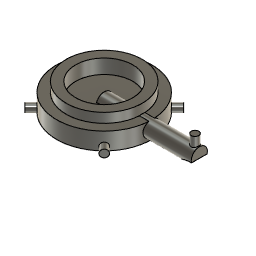
base v4 (Autodesk Fusion 360 design; units mm, degrees)
Autodesk Fusion 360 part; units mm, degrees
cylinder "CylinderPrimitive1" add diameter 100 height 8 placed x (1, 0, 0) y (0, 1, 0) z (0, 0, 1) at (0, 0, 0) makes body 1
cylinder "CylinderPrimitive2" add diameter 80 height 10 placed x (1, 0, 0) y (0, 1, 0) z (0, 0, 1) at (0, 0, 8) bodies 1
hole "Hole1" at (0, 0, 18) direction (0, 0, -1) diameter 60 depth 10 tip angle 180 bodies 1
cylinder "CylinderPrimitive3" add diameter 8 height 17 placed x (0, 1, 0) y (1, 0, 0) z (0, 0, -1) at (0, 0, 0) bodies 1
cylinder "CylinderPrimitive4" add diameter 8 height 10 placed x (0, 0, -1) y (0, 1, 0) z (1, 0, 0) at (0, 61, 25) separate body makes body 2
move_body "Move1" bodies 2 to x (1, 0, 0) y (0, 1, 0) z (0, 0, 1) at (50, -61, -21)
copy_body "CopyPasteBodies1" bodies 2 makes body 3
move_body "Move2" bodies 3 to x (1, 0, 0) y (0, 1, 0) z (0, 0, 1) at (-109, 0, 0)
move_body "Move3" bodies 2 to x (1, 0, 0) y (0, 1, 0) z (0, 0, 1) at (-1, 0, 0)
copy_body "CopyPasteBodies2" bodies 2 makes body 4
move_body "Move4" bodies 4 to x (0, 1, 0) y (-1, 0, 0) z (0, 0, 1) at (0, 0, 0)
copy_body "CopyPasteBodies3" bodies 3 makes body 5
move_body "Move5" bodies 5 to x (0, 1, 0) y (-1, 0, 0) z (0, 0, 1) at (0, 0, 0)
copy_body "CopyPasteBodies4" bodies 4 makes body 6
move_body "Move6" bodies 6 to x (0.707107, -0.707107, 0) y (0.707107, 0.707107, 0) z (0, 0, 1) at (0, 0, 0)
move_body "Move7" bodies 5 4 3 2 6 1 to x (0.707107, -0.707107, 0) y (0.707107, 0.707107, 0) z (0, 0, 1) at (0, 0, 0)
extrude "Extrude1" add 1 faces at (-0.8715, -0.8901, -17) along direction (0, 0, -1) blind 15 on bodies 1 bodies 1
extrude "Extrude2" add 1 faces at (59, 0.0132, 5.2456) along direction (1, 0, 0) blind 10 on bodies 6 bodies 6
extrude "Extrude3" add 1 faces at (69, 0.0132, 5.2456) along direction (1, 0, 0) blind 6 on bodies 6 bodies 6
extrude "Extrude4" add 1 faces at (75, 0.0132, 5.2456) along direction (1, 0, 0) blind 25 on bodies 6 bodies 6
hole "Hole2" at (100.1637, 0, -18.8091) direction (0, -1, 0) diameter 50 depth 60 tip angle 180 bodies 6
hole "Hole3" at (100.1637, 0, -18.8091) direction (0, 1, 0) diameter 50 depth 60 tip angle 180 bodies 6
cylinder "CylinderPrimitive5" add diameter 8 height 11 placed x (1, 0, 0) y (0, 1, 0) z (0, 0, 1) at (118.1372, 7.2715, 0) separate body makes body 7
move_body "Move8" bodies 7 to x (1, 0, 0) y (0, 1, 0) z (0, 0, 1) at (-23, 0, 7)
move_body "Move9" bodies 7 to x (1, 0, 0) y (0, 1, 0) z (0, 0, 1) at (0, -7, 0)
sketch "Sketch6" plane through (0, 0, 0) normal (1, 0, 0) x (0, 1, 0)
extrude "Extrude5" add 1 faces at (23.8686, -27.7358, 18) along direction (0, 0, 1) blind 10 on bodies 1 bodies 1
extrude "Extrude6" add 1 faces at (29.5997, -35.923, 8) along direction (0, 0, 1) blind 10 on bodies 1 bodies 1 7 2 3 4 5 6
move_body "Move10" bodies 7 to x (1, 0, 0) y (0, 1, 0) z (0, 0, 1) at (0, 0, 10)
cylinder "CylinderPrimitive6" add diameter 17 height 50 placed x (0, 0, -1) y (0, 1, 0) z (1, 0, 0) at (0, 0, 10) bodies 1
extrude "Extrude7" add 1 faces at (50, 0, 10.4062) along direction (1, 0, 0) blind 50 on bodies 1 bodies 1 7
extrude "Extrude8" add 1 faces at (-9.9734, 0.7289, 8) along direction (0, 0, 1) blind 5 on bodies 1 bodies 1
hole "Hole4" at (99.2078, 0, -12.1293) direction (0, -1, 0) diameter 40 depth 15 tip angle 118 bodies 1
hole "Hole5" at (99.2078, 0, -12.1293) direction (0, 1, 0) diameter 40 depth 38 tip angle 180 bodies 1
